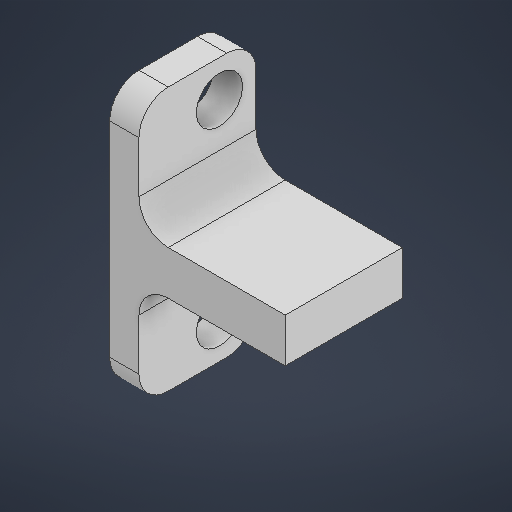
# Autodesk Inventor part: Uchwyt
Saved by Autodesk Inventor 2026 (Build 300175000, 175)
## iProperties
Created: 2025-04-27
Part Number: Uchwyt
Material: Generic
Document SubType Name: Modeling
Designer: isan
Density: 1 g/cm^3
Appearance: Default
Author: isan
Autodesk Inventor part; units mm, degrees
ref_plane "YZ Plane" through (0, 0, 0) normal (1, 0, 0) x (0, 1, 0)
ref_plane "XZ Plane" through (0, 0, 0) normal (0, 1, 0) x (-1, 0, 0)
ref_plane "XY Plane" through (0, 0, 0) normal (0, 0, 1) x (1, 0, 0)
sketch "Sketch1" plane through (0, 0, 0) normal (0, 1, 0) x (-1, 0, 0)
  line L0 (-1, 9) -> (1, 9)
  line L1 (1, 9) -> (1, -9)
  line L2 (1, -9) -> (-1, -9)
  line L3 (-1, -9) -> (-1, 9)
  line L4 (-1, 9) -> (1, -9) construction
  line L5 (1, 9) -> (-1, -9) construction
  point P0 (0, 0)
  dimension "d0" = 18
  dimension "d1" = 2
  constraints: 12 end point, 2 midpoint, 2 parallel, 1 horizontal, 1 perpendicular
  measures "d0" distance of L0.end L1.end
  measures "d1" distance of L1.end L2.end
extrude "Extrusion1" add sketch "Sketch1" along normal blind 8
fillet "Fillet1" radius 2 2 edges at (0, 8, 9) (0, 8, -9)
sketch "Sketch2" plane through (1, 0, 9) normal (1, 0, 0) x (0, 0, -1)
  circle A0 centre (2.5, 5.5) radius 1.575
  circle A1 centre (15.5, 5.5) radius 1.575
  line L0 (2, 8) -> (16, 8) projected
  line L1 (18, 0) -> (18, 6) projected
  line L2 (0, 0) -> (0, 6) projected
  point P0 (9, 0)
  point P1 (0, 3)
  dimension "d5" = 3.15
  dimension "d6" = 3.15
  dimension "d7" = 2.5
  dimension "d8" = 2.5
  dimension "d9" = 2.5
  dimension "d10" = 2.5
  constraints: 2 centre point, 1 midpoint
  measures "d5" diameter of A0
  measures "d6" diameter of A1
  measures "d7" distance from line of L0 A1.centre
  measures "d8" distance from line of L1 A1.centre
  measures "d9" distance from line of L0 A0.centre
  measures "d10" horizontal distance of point (0, 3) A0.centre
extrude "Extrusion2" cut sketch "Sketch2" against normal blind 2
fillet "Fillet2" radius 2 2 edges at (0, 0, 9) (0, 0, -9)
sketch "Sketch5" plane through (1, 8, 7) normal (1, 0, 0) x (0, 0, -1)
  line L0 (5.5, -8) -> (8.5, -8)
  line L1 (8.5, -8) -> (8.5, 0)
  line L2 (8.5, 0) -> (5.5, 0)
  line L3 (5.5, 0) -> (5.5, -8)
  line L4 (5.5, -8) -> (8.5, 0) construction
  line L5 (8.5, -8) -> (5.5, 0) construction
  line L6 (0, 0) -> (14, 0) projected
  line L7 (0, -8) -> (14, -8) projected
  line L8 (7, 0) -> (7, -8) construction
  line L9 (-2, -6) -> (-2, -2) projected
  line L10 (-2, -4) -> (16, -4) construction
  line L11 (16, -6) -> (16, -2) projected
  point P0 (7, -4)
  dimension "d14" = 3
  constraints: 16 end point, 6 midpoint, 2 collinear, 2 parallel, 2 perpendicular, 1 horizontal
  measures "d14" distance of L1.end L2.end
extrude "Extrusion3" add sketch "Sketch5" along normal blind 10
fillet "Face Fillet1" radius 2 1 edges at (1, 4, 1.5)
fillet "Face Fillet2" radius 2 1 edges at (1, 4, -1.5)
body "Solid1"
